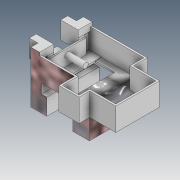
# Autodesk Inventor part: Peça1,61
Saved by Autodesk Inventor 2021 (Build 250183000, 183)
## iProperties
Created: 2020-10-08
Part Number: Peça1,61
Material: Genérico
Document SubType Name: Modeling
Designer: evert
Density: 1 g/cm^3
Appearance: Padrão
Author: evert
Autodesk Inventor part; units mm, degrees
ref_plane "YZ Plane" through (0, 0, 0) normal (1, 0, 0) x (0, 1, 0)
ref_plane "XZ Plane" through (0, 0, 0) normal (0, 1, 0) x (-1, 0, 0)
ref_plane "XY Plane" through (0, 0, 0) normal (0, 0, 1) x (1, 0, 0)
sketch "Esboço2" plane through (0, 0, 0) normal (0, 0, 1) x (1, 0, 0)
  line L0 (0, 0) -> (-5, 0)
  line L1 (-5, 0) -> (-5, -5)
  line L2 (-5, -5) -> (-2, -5)
  line L3 (-2, -5) -> (-2, -15)
  line L4 (-2, -15) -> (-5.6275, -15)
  line L5 (-5.6275, -15) -> (-5.6275, -20)
  line L6 (-5.6275, -20) -> (0, -20)
  line L7 (0, -20) -> (0, -17.5)
  line L8 (0, -17.5) -> (10, -17.5)
  line L9 (10, -17.5) -> (10, -20)
  line L10 (10, -20) -> (15, -20)
  line L11 (15, -20) -> (15, -15)
  line L12 (15, -15) -> (12.5, -15)
  line L13 (12.5, -15) -> (12.5, -5)
  line L14 (12.5, -5) -> (15, -5)
  line L15 (15, 0) -> (15, -5)
  line L16 (15, 0) -> (10, 0)
  line L17 (10, 0) -> (10, -2.5)
  line L18 (10, -2.5) -> (0, -2.5)
  line L19 (0, -2.5) -> (0, 0)
  line L20 (-2.2, -14.8) -> (-2.2, -5.2)
  line L21 (-2.2, -5.2) -> (-4.7, -5.2)
  line L22 (-2.2, -14.8) -> (-4.7, -14.8)
  line L23 (-2.2, -14.8) -> (-5.8275, -14.8)
  line L24 (-5.8275, -14.8) -> (-5.8275, -20)
  line L25 (-5.8275, -20) -> (-5.8275, -20.2)
  line L26 (-5.8275, -20.2) -> (0.2, -20.2)
  line L27 (0.2, -20.2) -> (0.2, -17.7)
  line L28 (0.2, -17.7) -> (9.8, -17.7)
  line L29 (9.8, -17.7) -> (9.8, -18.4636)
  line L30 (9.8, -18.4636) -> (9.8, -20.2)
  line L31 (9.8, -20.2) -> (15.2, -20.2)
  line L32 (15.2, -20.2) -> (15.2, -14.8)
  line L33 (15.2, -14.8) -> (12.7, -14.8)
  line L34 (12.7, -14.8) -> (12.7, -5.2)
  line L35 (12.7, -5.2) -> (15.1265, -5.2)
  line L36 (15.1265, -5.2) -> (15.2, -5.2)
  line L37 (15.2, -5.2) -> (15.2, 0)
  line L38 (-4.7, -5.2) -> (-5.2, -5.2)
  line L39 (-5.2, -5.2) -> (-5.2, 0)
  line L40 (-12.2, 0) -> (-12.2, -24.2)
  line L41 (-12.2, -24.2) -> (22.2, -24.2)
  line L42 (22.2, -24.2) -> (22.2, 0)
  line L43 (15.2, 0) -> (15.2, 0.2)
  line L44 (15.2, 0.2) -> (13.2, 0.2)
  line L45 (22.2, 0) -> (22.2, 1)
  line L46 (22.2, 1) -> (13.2, 1)
  line L47 (13.2, 1) -> (13.2, 0.2)
  line L48 (-12.2, 0) -> (-12.2, 1.2)
  line L49 (-5.2, 0) -> (-5.2, 0.2)
  line L50 (-5.2, 0.2) -> (-3.2, 0.2)
  line L51 (-3.2, 1.2) -> (-12.2, 1.2)
  line L52 (-3.2, 1.2) -> (0, 1.2)
  line L53 (0, 1.2) -> (0, 0.2)
  line L54 (0, 0.2) -> (-3.2, 0.2)
  line L55 (0.5946, -2.5) -> (0.5946, 9.5)
  line L56 (0.5946, 9.5) -> (9.5946, 9.5)
  line L57 (9.5946, 9.5) -> (9.5946, -2.5)
  line L58 (0.5946, -2.5) -> (9.5946, -2.5)
  dimension "d0" = 5
  dimension "d1" = 5
  dimension "d2" = 3
  dimension "d3" = 10
  dimension "d4" = 5
  dimension "d5" = 2.5
  dimension "d6" = 10
  dimension "d7" = 5
  dimension "d8" = 5
  dimension "d9" = 10
  dimension "d11" = 5
  dimension "d12" = 0.2
  dimension "d13" = 0.2
  dimension "d14" = 0.2
  dimension "d15" = 0.2
  dimension "d16" = 0.2
  dimension "d17" = 0.2
  dimension "d19" = 0.2
  dimension "d20" = 0.2
  dimension "d21" = 0.2
  dimension "d22" = 0.2
  dimension "d23" = 0.2
  dimension "d24" = 0.2
  dimension "d25" = 0.2
  dimension "d26" = 0.2
  dimension "d27" = 0.2
  dimension "d28" = 7
  dimension "d29" = 4
  dimension "d30" = 7
  dimension "d31" = 0.2
  dimension "d32" = 2
  dimension "d33" = 1
  dimension "d34" = 0.2
  dimension "d35" = 2
  dimension "d36" = 1
  dimension "d39" = 12
  dimension "d40" = 9
  constraints: 118 end point, 27 perpendicular, 16 point on line, 9 horizontal, 8 vertical, 3 parallel, 1 collinear
  measures "d0" distance of L0.start L0.end
  measures "d1" distance of L0.end L1.end
  measures "d2" distance of L1.end L2.end
  measures "d3" distance of L2.end L3.end
  measures "d4" distance of L4.end L5.end
  measures "d5" distance of L6.end L7.end
  measures "d6" distance of L7.end L8.end
  measures "d7" distance of L9.end L10.end
  measures "d8" distance of L10.end L11.end
  measures "d9" distance of L12.end L13.end
  measures "d11" distance of L15.start L16.end
  measures "d12" distance between parallel lines of L3 L20
  measures "d13" distance between parallel lines of L21 L2
  measures "d14" distance between parallel lines of L4 L22
  measures "d15" distance between parallel lines of L5 L24
  measures "d16" distance between parallel lines of L6 L26
  measures "d17" distance between parallel lines of L7 L27
  measures "d19" distance between parallel lines of L8 L28
  measures "d20" distance between parallel lines of L9 L29
  measures "d21" distance between parallel lines of L31 L10
  measures "d22" distance between parallel lines of L11 L32
  measures "d23" distance between parallel lines of L12 L33
  measures "d24" distance between parallel lines of L34 L13
  measures "d25" distance between parallel lines of L35 L14
  measures "d26" distance between parallel lines of L37 L15
  measures "d27" distance between parallel lines of L1 L39
  measures "d28" distance of L39.end L40.start
  measures "d29" distance from line of L41 L25.end
  measures "d30" distance from line of L42 L31.end
  measures "d31" distance of L37.end L43.end
  measures "d32" distance of L43.end L44.end
  measures "d33" distance of L42.end L45.end
  measures "d34" distance of L39.end L49.end
  measures "d35" distance of L49.end L50.end
  measures "d36" distance between parallel lines of L50 L51
  measures "d39" distance of L55.start L55.end
  measures "d40" distance of L55.end L56.end
extrude "Extrusão1" add sketch "Esboço2" along normal blind 30 contours L22 L23 L24 L25 L26 L27 L28 L29 L30 L31 L32 L33 L34 L35 L36 L37 L43 L44 L47 L46 L45 L42 L41 L40 L48 L51 L52 L53 L54 L50 L49 L39 L38 L21 L20
sketch "Esboço4" plane through (-12.2, -24.2, 0) normal (-1, 0, 0) x (0, 0, 1)
  circle A0 centre (30, 27.7) radius 6 projected
  line L0 (30, 27.7) -> (0, 27.7)
  line L1 (15, 27.7) -> (15, 25.4)
  line L2 (0, 25.4) -> (30, 25.4) projected
  line L3 (0, 27.7) -> (30, 27.7)
  line L4 (30, 27.7) -> (30, 25.4)
  line L5 (30, 25.4) -> (0, 25.4)
  line L6 (0, 25.4) -> (0, 27.7)
  point P0 (0, 24.2)
  constraints: 12 end point, 2 horizontal, 2 midpoint, 2 parallel, 1 perpendicular
extrude "Extrusão2" add sketch "Esboço4" against normal blind 5 contours L0 L4 L2 A0 | A0 L2 L1 L0 | L1 L2 L6 L0 picked at (28.1528, 26.1667)
sketch "Esboço5" plane through (-7.2, -24.2, 0) normal (1, 0, 0) x (0, 0, -1)
  line L0 (-30, 27.7) -> (0, 27.7) projected
  line L1 (0, 27.7) -> (-15, 27.7)
  circle A0 centre (-15, 27.7) radius 1.5
  point P0 (0, 24.2)
  dimension "d48" = 3
  constraints: 2 end point, 1 centre point, 1 coincident, 1 midpoint
  measures "d48" diameter of A0
extrude "Extrusão3" add sketch "Esboço5" along normal blind 13.7
sketch "Esboço6" plane through (-7.2, -24.2, 0) normal (-1, 0, 0) x (0, 0, 1)
  line L0 (13.5, 27.7) -> (16.5, 27.7) projected
  circle A0 centre (15, 27.7) radius 1.5
  point P0 (0, 24.2)
  constraints: 1 centre point, 1 midpoint
extrude "Extrusão4" add sketch "Esboço6" along normal blind 5 contours A0 L0 picked at (15.4855, 27.8197)
sketch "Esboço7" plane through (-12.2, -24.2, 0) normal (-1, 0, 0) x (0, 0, 1)
  circle A0 centre (30, 27.7) radius 6 projected
  line L0 (13.5, 27.7) -> (0, 27.7) projected
  line L1 (30, 33.7) -> (0, 33.7)
  line L2 (0, 33.7) -> (0, 27.7)
  line L3 (0, 27.7) -> (30, 27.7)
  line L4 (30, 27.7) -> (30, 33.7)
  point P0 (0, 24.2)
  constraints: 8 end point, 2 parallel, 1 horizontal, 1 perpendicular, 1 vertical alignment, 1 other
extrude "Extrusão5" add sketch "Esboço7" against normal blind 5 contours L4 L3 A0 | A0 L3 L0 L2 L1 picked at (26.0501, 28.145)
sketch "Esboço8" plane through (-12.2, -24.2, 0) normal (-1, 0, 0) x (0, 0, 1)
  line L0 (30, 33.7) -> (0, 33.7) projected
  line L1 (0, 33.7) -> (0, 35.2)
  line L2 (0, 35.2) -> (30, 35.2)
  line L3 (30, 35.2) -> (30, 33.7)
  line L4 (30, 33.7) -> (0, 33.7)
  line L5 (30, 33.7) -> (30, 25.4) projected
  point P0 (0, 24.2)
  dimension "d55" = 1.5
  constraints: 8 end point, 3 perpendicular, 1 vertical
  measures "d55" distance of L0.end L1.end
extrude "Extrusão6" add sketch "Esboço8" against normal blind 5
sketch "Esboço10" plane through (13.2, 1, 0) normal (0, 1, 0) x (1, 0, 0)
  line L0 (-6.7, -16.5) -> (-6.7, -13.5) projected
  line L1 (-6.7, -15) -> (-6.7, -21.5)
  line L2 (-6.7, -15) -> (-6.7, -8.5)
  line L3 (0, 0) -> (0, -30) projected
  line L4 (0, 0) -> (-13.2, 0)
  line L5 (-3.4, 0) -> (-13, 0) projected
  line L6 (-13.2, 0) -> (-13.2, -8.5)
  line L7 (-13, 0) -> (-13, -30) projected
  line L8 (-13.2, -8.5) -> (0, -8.5)
  line L9 (0, -8.5) -> (0, 0)
  line L10 (2, -30) -> (-3.4, -30) projected
  line L11 (0, -30) -> (0, -21.5)
  line L12 (0, -21.5) -> (-13.2, -21.5)
  line L13 (-13.2, 0) -> (-13.2, -30) projected
  line L14 (-13.2, -21.5) -> (-13.2, -30)
  line L15 (-13.2, -30) -> (0, -30)
  dimension "d58" = 6.5
  dimension "d59" = 6.5
  constraints: 20 end point, 5 perpendicular, 5 point on line, 2 collinear, 1 midpoint, 1 parallel
  measures "d58" distance of L1.start L1.end
  measures "d59" distance of L1.start L2.end
extrude "Extrusão7" add sketch "Esboço10" against normal blind 0.8 contours L12 L3 L10 L15 L7 | L7 L15 L13 L12 | L8 L7 L4 L3 | L8 L6 L4 L7
sketch "Esboço15" plane through (22.2, -24.2, 0) normal (1, 0, 0) x (0, 0, -1)
  line L0 (-30, 25.2) -> (-21.5, 25.2) projected
  line L1 (-30, 25.2) -> (0, 25.2)
  line L2 (0, 25.2) -> (0, 24.2)
  line L3 (0, 24.2) -> (-30, 24.2)
  line L4 (-30, 24.2) -> (-30, 25.2)
  constraints: 8 end point, 2 parallel, 1 horizontal, 1 perpendicular
extrude "Extrusão10" add sketch "Esboço15" along normal blind 3
sketch "Esboço16" plane through (0, 1, 8.5) normal (0, 1, 0) x (1, 0, 0)
  line L0 (22.2, -21.5) -> (25.2, -21.5) projected
  line L1 (25.2, 8.5) -> (23.7, 8.5)
  line L2 (23.7, -21.5) -> (25.2, -21.5)
  line L3 (0, -21.5) -> (25.2, -21.5) projected
  line L4 (-12.2, -21.5) -> (-12.2, 8.5) projected
  line L5 (25.2, -21.5) -> (-12.2, -21.5)
  line L6 (-12.2, -21.5) -> (-12.2, -20.5)
  line L7 (-12.2, -20.5) -> (25.2, -20.5)
  line L8 (25.2, -20.5) -> (25.2, -21.5)
  line L9 (0, 8.5) -> (25.2, 8.5) projected
  line L10 (25.2, 8.5) -> (-12.2, 8.5)
  line L11 (-12.2, 8.5) -> (-12.2, 7.5)
  line L12 (-12.2, 7.5) -> (25.2, 7.5)
  line L13 (25.2, 7.5) -> (25.2, 8.5)
  line L14 (25.2, 8.5) -> (24.2, 8.5)
  line L15 (24.2, 8.5) -> (24.2, -21.5)
  line L16 (24.2, -21.5) -> (25.2, -21.5)
  line L17 (25.2, -21.5) -> (25.2, 8.5)
  point P0 (24.2, 7.5)
  point P1 (24.2, -20.5)
  dimension "d70" = 1
  dimension "d71" = 1
  dimension "d73" = 1
  constraints: 28 end point, 7 parallel, 4 horizontal, 3 perpendicular, 3 point on line, 1 midpoint
  measures "d70" distance between parallel lines of L9 L12
  measures "d71" distance between parallel lines of L7 L3
  measures "d73" distance of L16.end L15.end
extrude "Extrusão11" add sketch "Esboço16" along normal blind 10 contours L3 L5 L4 L7 L15 L0 | L15 L7 L8 L0 | L15 L12 L17 L7 | L15 L1 L13 L12 | L12 L4 L10 L9 L1 L15
sketch "Esboço18" plane through (0, 0, 30) normal (0, 0, 1) x (1, 0, 0)
  line L0 (-12.2, 11) -> (-12.2, -24.2) projected
  line L1 (-12.2, -24.2) -> (22.2, -24.2) projected
  line L2 (-12.2, 11) -> (-11.2, 11)
  line L3 (-11.2, 11) -> (-11.2, -24.2)
  line L4 (-11.2, -24.2) -> (-12.2, -24.2)
  line L5 (-12.2, -24.2) -> (-12.2, 11)
  point P0 (0, 0)
  dimension "d76" = 1
  constraints: 8 end point, 2 parallel, 1 horizontal, 1 perpendicular, 1 point on line
  measures "d76" distance of L3.end L4.end
extrude "Extrusão12" cut sketch "Esboço18" against normal through all
sketch "Esboço20" plane through (0, 1, 8.5) normal (0, 1, 0) x (1, 0, 0)
  line L0 (0, 7.5) -> (0, -20.5) projected
  line L1 (12.7, 8.5) -> (12.7, -21.5) projected
  line L2 (0, 0) -> (12.7, 0)
  line L3 (12.7, 0) -> (12.7, 1)
  line L4 (12.7, 1) -> (0, 1)
  line L5 (0, 1) -> (0, 0)
  line L6 (0, 0) -> (13.2, 0) projected
  line L7 (12.7, 1) -> (13.2, 1)
  line L8 (13.2, 1) -> (13.2, 0)
  line L9 (13.2, 0) -> (12.7, 0)
  line L10 (12.7, 0) -> (12.7, 1)
  line L11 (13.2, 0) -> (13.2, -13) projected
  line L12 (0, -20.5) -> (0, -13) projected
  line L13 (13.2, -13) -> (0, -13)
  line L14 (0, -13) -> (0, -14)
  line L15 (0, -14) -> (13.2, -14)
  line L16 (13.2, -14) -> (13.2, -13)
  point P0 (0, 8.5)
  point P1 (0, -14)
  point P2 (0, -13)
  point P3 (0, 1)
  dimension "d79" = 1
  dimension "d80" = 1
  constraints: 24 end point, 6 parallel, 3 horizontal, 3 perpendicular, 3 point on line
  measures "d79" distance between parallel lines of L4 L2
  measures "d80" distance between parallel lines of L15 L13
extrude "Extrusão13" cut sketch "Esboço20" against normal blind 1 contours L4 L1 L2 L0 | L7 L8 L6 L1 | L13 L1 L15 L0 | L13 L16 L15 L1
sketch "Esboço23" plane through (0, 1, 29) normal (0, 1, 0) x (1, 0, 0)
  line L0 (13.2, 21.5) -> (13.2, 6.5) projected
  line L1 (13.2, 6.5) -> (17.9377, 6.5)
  line L2 (17.9377, 6.5) -> (22.2, 6.5)
  line L3 (22.2, 29) -> (22.2, -1) projected
  line L4 (13.2, 6.5) -> (23.7, 6.5)
  line L5 (13.2, 21.5) -> (0, 21.5) projected
  line L6 (13.2, 21.5) -> (23.7, 21.5)
  line L7 (13.2, 21.5) -> (13.2, 6.5)
  line L8 (23.7, 6.5) -> (23.7, 21.5)
  point P0 (0, 29)
  point P1 (22.2, 21.5)
  point P2 (22.2, 6.5)
  dimension "d91" = 10.5
  constraints: 12 end point, 3 point on line, 2 equal length, 1 horizontal, 1 perpendicular
  measures "d91" distance of L0.end L4.end
extrude "Extrusão16" cut sketch "Esboço23" against normal blind 0.5
sketch "Esboço29" plane through (0, 0.5, 29) normal (0, 1, 0) x (1, 0, 0)
  line L0 (13.2, 6.5) -> (13.2, 21.5) projected
  line L1 (13.2, 21.5) -> (10.2, 21.5)
  line L2 (0, 21.5) -> (23.7, 21.5) projected
  line L3 (10.2, 21.5) -> (10.2, 6.5)
  line L4 (23.7, 6.5) -> (0, 6.5) projected
  line L5 (13.2, 6.5) -> (10.2, 6.5)
  line L6 (10.2, 21.5) -> (13.2, 21.5)
  point P0 (0, 29)
  dimension "d102" = 3
  constraints: 8 end point, 2 perpendicular, 2 point on line, 1 collinear
  measures "d102" distance of L0.end L1.end
extrude "Extrusão20" add sketch "Esboço29" against normal blind 0.5
sketch "Esboço38" plane through (-11.2, -24.2, 30) normal (-1, 0, 0) x (0, 0, 1)
  line L0 (0, 35.2) -> (0, 0) projected
  line L1 (-30, 24.2) -> (0, 24.2) projected
  line L2 (0, 24.2) -> (-30, 24.2)
  line L3 (-30, 35.2) -> (0, 35.2) projected
  line L4 (-25, 35.2) -> (-25, 24.2)
  line L5 (-5, 35.2) -> (-5, 24.2)
  line L6 (-5, 24.2) -> (-10, 24.2)
  line L7 (-7.5, 24.2) -> (-22.5, 24.2) projected
  line L8 (-10, 24.2) -> (-10, 27.2)
  line L9 (-10, 27.2) -> (-20, 27.2)
  line L10 (-20, 27.2) -> (-20, 24.2)
  line L11 (-5, 24.2) -> (-5, 29.2)
  line L12 (-5, 29.2) -> (-8, 29.2)
  line L13 (-8, 29.2) -> (-8, 35.2)
  line L14 (-25, 24.2) -> (-25, 29.2)
  line L15 (-25, 29.2) -> (-22, 29.2)
  line L16 (-22, 29.2) -> (-22, 35.2)
  line L17 (-22, 35.2) -> (-8, 35.2)
  point P0 (-5, 24.2)
  dimension "d128" = 20
  dimension "d129" = 5
  dimension "d130" = 5
  dimension "d131" = 3
  dimension "d132" = 10
  dimension "d133" = 5
  dimension "d134" = 3
  dimension "d135" = 3
  constraints: 28 end point, 12 point on line, 7 perpendicular, 2 collinear, 1 vertical
  measures "d128" distance between parallel lines of L5 L4
  measures "d129" distance between parallel lines of L0 L5
  measures "d130" distance of L5.end L6.end
  measures "d131" distance of L6.end L8.end
  measures "d132" distance of L8.end L9.end
  measures "d133" distance of L5.end L11.end
  measures "d134" distance of L11.end L12.end
  measures "d135" distance of L14.end L15.end
extrude "Extrusão25" cut sketch "Esboço38" against normal blind 5 contours L1 L8 L9 L10 L4 L15 L16 L3 L13 L12 L5
sketch "Esboço39" plane through (-7.2, 1.2, 29) normal (0, 1, 0) x (1, 0, 0)
  line L0 (1, 12.5) -> (13.7, 12.5) projected
  line L1 (1, 12.5) -> (1, 4)
  line L2 (1, 4) -> (0, 4) projected
  line L3 (1, 4) -> (0, 4)
  line L4 (1, 24) -> (1, 19) projected
  line L5 (1, 12.5) -> (1, 24)
  line L6 (1, 24) -> (0, 24)
  line L7 (0, 24) -> (0, 24.1)
  line L8 (0, 28) -> (0, 21) projected
  line L9 (0, 24.1) -> (1.1, 24.1)
  line L10 (0, 4) -> (0, 0) projected
  line L11 (0, 4) -> (0, 3.9)
  line L12 (0, 3.9) -> (1.1, 3.9)
  line L13 (1.1, 3.9) -> (1.1, 24.1)
  point P0 (7.2, 29)
  dimension "d138" = 0.1
  dimension "d139" = 1.1
  dimension "d140" = 0.1
  constraints: 18 end point, 3 point on line, 2 collinear, 2 parallel, 2 perpendicular, 1 vertical
  measures "d138" distance of L6.end L7.end
  measures "d139" distance of L7.end L9.end
  measures "d140" distance of L2.end L11.end
extrude "Extrusão26" add sketch "Esboço39" along normal blind 9.8
sketch "Esboço40" plane through (-11.2, 3, 20) normal (0, 1, 0) x (1, 0, 0)
  line L0 (4, 3.5858) -> (4, 0) projected
  line L1 (5, 3.5858) -> (4, 3.5858) projected
  line L2 (4, 0) -> (5, 0)
  line L3 (5, 0) -> (5, 3.5858)
  line L4 (5, 3.5858) -> (4, 3.5858)
  line L5 (4, 3.5858) -> (4, 0)
  line L6 (4, 6.4142) -> (5, 6.4142) projected
  line L7 (4, 6.4142) -> (5, 6.4142)
  line L8 (5, 6.4142) -> (5, 10)
  line L9 (5, 10) -> (4, 10)
  line L10 (4, 10) -> (4, 6.4142)
  point P0 (11.2, 20)
  constraints: 16 end point, 4 parallel, 2 horizontal, 2 perpendicular
extrude "Extrusão27" add sketch "Esboço40" against normal blind 10
sketch "Esboço41" plane through (-7.2, 1.2, 29) normal (0, 1, 0) x (1, 0, 0)
  line L0 (1, 19) -> (1, 15.4142) projected
  line L1 (1, 19) -> (1.8, 19)
  line L2 (1.3725, 29) -> (1.3725, -1) projected
  line L3 (1, 24) -> (1, 4) projected
  line L4 (1, 9.0006) -> (1.8, 9.0006)
  line L5 (1.8, 19) -> (1.8, 9.0006)
  line L6 (1.8, 9.0006) -> (1.8, 3.2006)
  line L7 (1.8, 3.2006) -> (0, 3.2006)
  line L8 (1.8, 19) -> (1.8, 24.8)
  line L9 (1.8, 24.8) -> (0, 24.8)
  line L10 (0, 28) -> (0, 24.1) projected
  line L11 (0, 24.8) -> (0, 24.1)
  line L12 (1.1, 24.1) -> (0, 24.1) projected
  line L13 (0, 24.1) -> (1.1, 24.1)
  line L14 (0, 3.9) -> (0, 0) projected
  line L15 (0, 3.2006) -> (0, 3.9)
  line L16 (0, 3.9) -> (1.1, 3.9) projected
  line L17 (0, 3.9) -> (1.1, 3.9)
  line L18 (1.1, 3.9) -> (1.1, 9.0006)
  line L19 (1.1, 3.9) -> (1.1, 24.1) projected
  line L20 (1.1, 3.9) -> (1.1, 24.1)
  line L21 (0, 28) -> (0, 24.1) projected
  line L22 (0, 24.1) -> (1.1, 24.1)
  line L23 (0, 24.1) -> (0, 24.8)
  point P0 (7.2, 29)
  point P1 (1.1, 19)
  dimension "d149" = 5.8
  dimension "d150" = 5.8
  constraints: 30 end point, 6 perpendicular, 4 collinear, 3 point on line, 3 vertical, 1 horizontal
  measures "d149" distance of L4.end L6.end
  measures "d150" distance of L1.end L8.end
extrude "Extrusão28" add sketch "Esboço41" along normal blind 9.8
sketch "Esboço42" plane through (-7.2, -24.2, 0) normal (1, 0, 0) x (0, 0, -1)
  line L0 (-22, 35.2) -> (-25, 35.2) projected
  line L1 (-22, 35.2) -> (-22, 29.2)
  line L2 (-22, 29.2) -> (-25, 29.1118)
  line L3 (-25, 25.4) -> (-25, 35.2) projected
  line L4 (-25, 35.2) -> (-25, 35.2) projected
  line L5 (-25, 29.2) -> (-22, 29.2) projected
  line L6 (-25, 35.2) -> (-25, 29.2)
  line L7 (-22, 29.2) -> (-22, 35.2) projected
  line L8 (-25, 35.2) -> (-22, 35.2)
  point P0 (0, 24.2)
  constraints: 8 end point, 1 horizontal, 1 perpendicular, 1 point on line
extrude "Extrusão29" add sketch "Esboço42" along normal blind 1.5 contours L1 L5 L3 L0
sketch "Esboço43" plane through (-7.2, -24.2, 0) normal (1, 0, 0) x (0, 0, -1)
  line L0 (-5, 35.2) -> (-5, 35.4) projected
  line L1 (-8, 35.2) -> (-5, 35.2)
  line L2 (-5, 35.2) -> (-8, 35.2) projected
  line L3 (-8, 35.2) -> (-7.9375, 31.75)
  line L4 (-8, 35.2) -> (-8, 29.2086)
  line L5 (-8, 29.2086) -> (-5, 29.2)
  line L6 (-5, 29.2) -> (-5, 35.2)
  point P0 (0, 24.2)
  constraints: 10 end point, 1 collinear, 1 horizontal, 1 vertical
extrude "Extrusão30" add sketch "Esboço43" along normal blind 1.5
sketch "Esboço44" plane through (-11.2, -24.2, 30) normal (-1, 0, 0) x (0, 0, 1)
  line L0 (-7.5, 24.2) -> (-22.5, 24.2) projected
  line L1 (-20, 27.2) -> (-9.9695, 27.2)
  line L2 (-9.9695, 27.2) -> (-9.9695, 24.2)
  line L3 (-9.9695, 24.2) -> (-20, 24.2)
  line L4 (-20, 24.2) -> (-20, 27.2)
  point P0 (-30, 24.2)
  constraints: 8 end point, 2 parallel, 1 horizontal, 1 perpendicular, 1 point on line
extrude "Extrusão31" add sketch "Esboço44" along normal blind 5
sketch "Esboço45" plane through (-11.2, -24.2, 30) normal (-1, 0, 0) x (0, 0, 1)
  line L0 (-8, 35.2) -> (-8, 29.2) projected
  line L1 (-8, 29.2) -> (-8, 39.2)
  line L2 (-8, 39.2) -> (0, 39.2)
  line L3 (-8, 35.2) -> (0, 35.2) projected
  line L4 (0, 39.2) -> (0, 35.2)
  line L5 (0, 35.2) -> (-8, 35.2)
  line L6 (-30, 35.2) -> (-22, 35.2) projected
  line L7 (-22, 35.2) -> (-22, 39.2)
  line L8 (-22, 39.2) -> (-30, 39.2)
  line L9 (-30, 39.2) -> (-30, 35.2)
  line L10 (-8, 29.2) -> (-5, 29.2) projected
  line L11 (-8, 29.2) -> (0, 29.2)
  line L12 (0, 29.2) -> (0, 39.2)
  line L13 (-22, 35.2) -> (-22, 29.2086) projected
  line L14 (-22, 35.2) -> (-22, 29.2086)
  line L15 (-22, 29.2086) -> (-30, 29.2)
  line L16 (-30, 0) -> (-30, 35.2) projected
  line L17 (-30, 39.2) -> (-30, 29.2)
  point P0 (-30, 24.2)
  dimension "d157" = 10
  constraints: 24 end point, 4 collinear, 3 perpendicular, 2 horizontal, 2 point on line, 1 vertical
  measures "d157" distance of L0.end L1.end
extrude "Extrusão32" add sketch "Esboço45" along normal blind 5
sketch "Esboço46" plane through (-11.2, -24.2, 30) normal (1, 0, 0) x (0, 0, -1)
  line L0 (0, 39.2) -> (8, 39.2) projected
  line L1 (8, 39.2) -> (8, 35.2) projected
  line L2 (0, 39.2) -> (8, 39.2)
  line L3 (8, 39.2) -> (8, 35.2)
  line L4 (0, 35.2) -> (0, 39.2) projected
  line L5 (8, 35.2) -> (0, 35.2)
  line L6 (0, 35.2) -> (0, 39.2)
  line L7 (22, 29.2086) -> (22, 39.2) projected
  line L8 (22, 39.2) -> (30, 39.2)
  line L9 (30, 35.2) -> (22, 35.2) projected
  line L10 (30, 39.2) -> (30, 35.2)
  line L11 (30, 35.2) -> (22, 35.2)
  line L12 (22, 35.2) -> (22, 39.2)
  point P0 (30, 24.2)
  constraints: 16 end point, 3 collinear, 3 perpendicular, 2 horizontal
extrude "Extrusão33" add sketch "Esboço46" along normal blind 5
sketch "Esboço47" plane through (-16.2, -24.2, 30) normal (-1, 0, 0) x (0, 0, 1)
  line L0 (0, 29.2) -> (-5, 29.2) projected
  line L1 (-8, 29.2) -> (-5, 29.2)
  line L2 (-8, 29.2) -> (-4, 29.2)
  line L3 (-4, 29.2) -> (-4, 39.2)
  line L4 (0, 39.2) -> (-8, 39.2) projected
  line L5 (0, 39.2) -> (-4, 39.2)
  line L6 (0, 29.2) -> (0, 39.2) projected
  line L7 (0, 39.2) -> (0, 29.2)
  line L8 (0, 29.2) -> (-4, 29.2)
  line L9 (-25, 29.2) -> (-22, 29.2) projected
  line L10 (-22, 29.2) -> (-26, 29.2043)
  line L11 (-22, 29.2086) -> (-30, 29.2) projected
  line L12 (-26, 29.2043) -> (-26, 39.2)
  line L13 (-30, 39.2) -> (-22, 39.2) projected
  line L14 (-30, 39.2) -> (-26, 39.2)
  line L15 (-30, 35.2) -> (-30, 39.2) projected
  line L16 (-30, 39.2) -> (-30, 29.2086)
  line L17 (-30, 29.2086) -> (-26, 29.2043)
  point P0 (-30, 24.2)
  dimension "d163" = 4
  constraints: 22 end point, 5 collinear, 3 midpoint, 3 point on line, 1 perpendicular
  measures "d163" distance of L1.start L2.end
extrude "Extrusão34" cut sketch "Esboço47" against normal blind 5
sketch "Esboço48" plane through (-16.2, 5.0043, 4) normal (0, 1, 0.0011) x (1, 0, 0)
  line L0 (5, 4) -> (5, 4.0107) projected
  line L1 (5, 0) -> (5, 4) projected
  line L2 (5, 4.0107) -> (5, 0)
  line L3 (5, 0.0107) -> (0, 0.0107) projected
  line L4 (5, 0) -> (0, 0.0107)
  line L5 (0, 4) -> (5, 4) projected
  line L6 (0.0086, 4.0107) -> (5, 4.0107)
  line L7 (0, 0.0107) -> (0, 0) projected
  line L8 (0, 0) -> (-1.8529, 0)
  line L9 (-1.8529, 0) -> (-1.8529, 4)
  line L10 (-1.8529, 4) -> (0, 4)
  point P0 (16.2, 3.9946)
  constraints: 12 end point, 2 perpendicular, 1 horizontal, 1 vertical, 1 vertical alignment, 2 other
extrude "Extrusão35" cut sketch "Esboço48" against normal blind 5 contours L3 L7 L8 L9 L10 L5 L1
sketch "Esboço50" plane through (22.2, -24.2, 0) normal (0, -1, 0) x (1, 0, 0)
  line L0 (-28.4, 0) -> (-38.4, 0) projected
  line L1 (0, 30) -> (-33.4, 30)
  line L2 (-33.4, 30) -> (-33.4, 0)
  line L3 (-33.4, 0) -> (0, 0)
  line L4 (0, 0) -> (0, 30)
  point P0 (-22.2, 0)
  constraints: 8 end point, 2 parallel, 1 horizontal, 1 perpendicular
extrude "Extrusão36" cut sketch "Esboço50" against normal blind 9.5
sketch "Esboço51" plane through (25.2, 11, 30) normal (0, 1, 0) x (1, 0, 0)
  line L0 (-36.4, 0) -> (-27.4, 0) projected
  line L1 (-31.407, 0) -> (0, 0)
  line L2 (0, 0) -> (0, 30)
  line L3 (0, 30) -> (-31.407, 30)
  line L4 (-31.407, 30) -> (-31.407, 0)
  line L5 (0, 30) -> (-31.407, 30)
  line L6 (-31.407, 30) -> (-31.407, 50)
  line L7 (-31.407, 50) -> (0, 50)
  line L8 (0, 50) -> (0, 30)
  point P0 (-25.2, 30)
  dimension "d172" = 20
  constraints: 16 end point, 4 parallel, 2 horizontal, 2 perpendicular, 2 point on line
  measures "d172" distance of L5.end L6.end
extrude "Extrusão37" cut sketch "Esboço51" against normal blind 1.2 contours L4 L3 L2 L1 L0
sketch "Esboço52" plane through (0, 1, 29) normal (0, 1, 0) x (1, 0, 0)
  line L0 (10.2, 21.5) -> (13.2, 21.5) projected
  line L1 (10.2, 6.5) -> (10.2, 21.5) projected
  line L2 (10.2, 21.5) -> (10.2, 6.5)
  line L3 (13.2, 6.5) -> (10.2, 6.5) projected
  line L4 (10.2, 6.5) -> (10.2, 14)
  line L5 (10.2, 14) -> (0, 14)
  line L6 (0, 21.5) -> (0, 6.5) projected
  line L7 (10.2, 14) -> (10.2, 21.5)
  line L8 (10.2, 14) -> (10.2, 24.5)
  line L9 (10.2, 14) -> (10.2, 3.5)
  line L10 (10.2, 3.5) -> (0, 3.5)
  line L11 (0, 28) -> (0, 0) projected
  line L12 (0, 3.5) -> (0, 24.5)
  line L13 (0, 21.5) -> (0, 28) projected
  line L14 (0, 24.5) -> (10.2, 24.5)
  point P0 (0, 29)
  point P1 (10.2, 6.5)
  point P2 (10.2, 21.5)
  dimension "d175" = 10.5
  dimension "d176" = 10.5
  dimension "d177" = 21
  constraints: 18 end point, 3 point on line, 2 midpoint, 1 collinear, 1 perpendicular, 1 vertical
  measures "d175" distance of L4.end L8.end
  measures "d176" distance of L4.end L9.end
  measures "d177" distance of L10.end L12.end
extrude "Extrusão38" cut sketch "Esboço52" against normal blind 10
sketch "Esboço53" plane through (0, 0.5, 29) normal (0, 1, 0) x (1, 0, 0)
  line L0 (10.2, 6.5) -> (13.2, 6.5) projected
  line L1 (23.7, 21.5) -> (23.7, 6.5) projected
  line L2 (10.2, 6.5) -> (23.7, 6.5)
  line L3 (23.7, 6.5) -> (23.7, 21.5)
  line L4 (23.7, 21.5) -> (10.2, 21.5)
  line L5 (10.2, 21.5) -> (10.2, 6.5)
  point P0 (0, 29)
  point P1 (13.2, 6.5)
  constraints: 8 end point, 2 parallel, 1 horizontal, 1 perpendicular
extrude "Extrusão39" add sketch "Esboço53" along normal blind 0.5
sketch "Esboço56" plane through (25.2, 9.8, 30) normal (0, 1, 0) x (1, 0, 0)
  line L0 (0, 0) -> (-31.407, 0) projected
  line L1 (-12.5, 30) -> (-12.5, 0) projected
  line L2 (0, 0) -> (-12.5, 0)
  line L3 (-12.5, 0) -> (-12.5, 28.9999)
  line L4 (-12.5, 28.9999) -> (0, 28.9999)
  line L5 (0, 28.9999) -> (0, 0)
  point P0 (-25.2, 30)
  constraints: 8 end point, 2 parallel, 1 horizontal, 1 perpendicular, 1 point on line
extrude "Extrusão40" cut sketch "Esboço56" against normal blind 8.8
sketch "Esboço57" plane through (-5.4, 1.2, 25.7994) normal (1, 0, 0) x (0, 0, -1)
  circle A0 centre (10.7994, 2.3) radius 1.5 projected
  line L0 (10.7994, 0.8) -> (10.7994, 2.3)
  line L1 (10.7994, 2.3) -> (10.7994, 5.3)
  circle A1 centre (10.7994, 5.3) radius 1.5
  line L2 (12.2994, 2.3) -> (12.2994, 5.3)
  line L3 (9.2994, 2.3) -> (9.2994, 5.3)
  point P0 (25.7994, -1.2)
  dimension "d187" = 3
  dimension "d188" = 3
  constraints: 8 end point, 5 point on circle, 2 tangent, 2 vertical, 1 centre point, 1 coincident, 1 parallel, 1 point on line
  measures "d187" distance of L0.end L1.end
  measures "d188" diameter of A1
extrude "Extrusão41" add sketch "Esboço57" along normal blind 12.2 contours A1
sketch "Esboço58" plane through (6.5, 3.5, 15) normal (1, 0, 0) x (0, 0, -1)
  circle A0 centre (0, 0) radius 1.5
  point P0 (15, -3.5)
  constraints: 1 centre point
extrude "Extrusão42" cut sketch "Esboço58" against normal blind 11.9
sketch "Esboço59" plane through (0, 1, 1) normal (0, 1, 0) x (1, 0, 0)
  line L0 (10.2, -3.5) -> (10.2, -24.5) projected
  line L1 (10.2, -24.5) -> (11.2, -24.5)
  line L2 (11.2, -24.5) -> (11.2, -3.5)
  line L3 (11.2, -3.5) -> (10.2, -3.5)
  line L4 (10.2, -3.5) -> (10.2, -24.5)
  point P0 (0, 1)
  dimension "d193" = 1
  constraints: 8 end point, 2 parallel, 1 horizontal, 1 perpendicular
  measures "d193" distance of L2.end L3.end
extrude "Extrusão43" cut sketch "Esboço59" against normal blind 1
sketch "Esboço61" plane through (6.8, 6.5, 15) normal (1, 0, 0) x (0, 0, -1)
  circle A0 centre (0, 0) radius 1.5 projected
  circle A1 centre (0, 0) radius 1.5
  point P0 (15, -6.5)
  constraints: 1 centre point, 1 coincident
extrude "Extrusão44" cut sketch "Esboço61" against normal blind 1.8
sketch "Esboço62" plane through (25.2, 9.8, 30) normal (0, 1, 0) x (1, 0, 0)
  line L0 (-31.4, 30) -> (-31.4, 22) projected
  line L1 (-31.4, 29.0001) -> (-31.4, 30)
  line L2 (-31.4, 30) -> (0.1, 30)
  line L3 (0.1, 30) -> (0.1, 22.04)
  line L4 (0.1, 30) -> (-0.9, 30)
  line L5 (-3, 30) -> (0, 30) projected
  line L6 (-0.9, 30) -> (-0.9, 21.04)
  line L7 (-0.9, 21.04) -> (14, 21.04)
  line L8 (0.1, 22.04) -> (15, 22.04)
  line L9 (15, 22.04) -> (15, -2.96)
  line L10 (14, 21.04) -> (14, -1.96)
  line L11 (15, -2.96) -> (0.1, -2.96)
  line L12 (14, -1.96) -> (-0.9, -1.96)
  line L13 (-0.9, -1.96) -> (-0.9, -7.96)
  line L14 (0.1, -2.96) -> (0.1, -8.96)
  line L15 (0.1, -8.96) -> (-11.5, -8.96)
  line L16 (-0.9, -7.96) -> (-10.5, -7.96)
  line L17 (-11.5, -8.96) -> (-11.5, 1)
  line L18 (-10.5, -7.96) -> (-10.5, 1)
  line L19 (-10, 0) -> (-12.5, 0) projected
  line L20 (-25.2, 1) -> (-12.5, 1) projected
  line L21 (-10.5, 1) -> (-12.5, 1)
  line L22 (-12.5, 30) -> (-12.5, 0) projected
  line L23 (-12.5, 1) -> (-12.5, 0)
  line L24 (-12.5, 0) -> (-10.5, 0)
  point P0 (-25.2, 30)
  point P1 (-11.5, 0)
  point P2 (-0.9, 30)
  dimension "d198" = 31.5
  dimension "d199" = 7.96
  dimension "d200" = 1
  dimension "d201" = 8.96
  dimension "d202" = 14.9
  dimension "d203" = 14.9
  dimension "d204" = 25
  dimension "d205" = 23
  dimension "d206" = 14.9
  dimension "d207" = 14.9
  dimension "d208" = 6
  dimension "d209" = 6
  dimension "d210" = 11.6
  dimension "d211" = 9.6
  dimension "d212" = 9.96
  dimension "d213" = 8.96
  constraints: 40 end point, 7 horizontal, 7 vertical, 4 point on line, 1 collinear, 1 perpendicular
  measures "d198" distance of L0.start L2.end
  measures "d199" distance of L2.end L3.end
  measures "d200" distance of L2.end L4.end
  measures "d201" distance of L4.end L6.end
  measures "d202" distance of L6.end L7.end
  measures "d203" distance of L3.end L8.end
  measures "d204" distance of L8.end L9.end
  measures "d205" distance of L7.end L10.end
  measures "d206" distance of L9.end L11.end
  measures "d207" distance of L10.end L12.end
  measures "d208" distance of L12.end L13.end
  measures "d209" distance of L11.end L14.end
  measures "d210" distance of L14.end L15.end
  measures "d211" distance of L13.end L16.end
  measures "d212" distance of L15.end L17.end
  measures "d213" distance of L16.end L18.end
extrude "Extrusão45" add sketch "Esboço62" against normal blind 8.8 contours L21 L17 L19 L22 | L2 L3 L8 L9 L11 L14 L15 L17 L19 L18 L16 L13 L12 L10 L7 L6 | L21 L18 L19 L17
sketch "Esboço63" plane through (25.2, 9.8, 30) normal (0, 1, 0) x (1, 0, 0)
  line L0 (-31.4, 8) -> (-31.4, 0) projected
  line L1 (-31.407, 1) -> (-10.5, 1) projected
  line L2 (-31.4, 0) -> (-10.5, 0)
  line L3 (-10.5, 0) -> (-10.5, 1)
  line L4 (-10.5, 1) -> (-31.4, 1)
  line L5 (-31.4, 1) -> (-31.4, 0)
  line L6 (-11.5, 0) -> (-11.5, -8.96) projected
  line L7 (-10.5, 1) -> (-11.5, 1)
  line L8 (-11.5, 1) -> (-11.5, -8.96)
  line L9 (-11.5, -8.96) -> (-10.5, -8.96)
  line L10 (-10.5, -8.96) -> (-10.5, 1)
  line L11 (-11.5, -8.96) -> (0.1, -8.96) projected
  line L12 (-10.5, -7.96) -> (-0.9, -7.96) projected
  line L13 (-11.5, -8.96) -> (-0.9, -8.96)
  line L14 (-0.9, -8.96) -> (-0.9, -7.96)
  line L15 (-0.9, -7.96) -> (-11.5, -7.96)
  line L16 (-11.5, -7.96) -> (-11.5, -8.96)
  line L17 (-0.9, -1.96) -> (14, -1.96) projected
  line L18 (-0.9, -8.96) -> (0.1, -8.96)
  line L19 (0.1, -8.96) -> (0.1, -1.96)
  line L20 (0.1, -1.96) -> (-0.9, -1.96)
  line L21 (-0.9, -1.96) -> (-0.9, -8.96)
  line L22 (-0.9, -7.96) -> (-0.9, -1.96) projected
  line L23 (15, 22.04) -> (15, -2.96) projected
  line L24 (-0.9, -1.96) -> (15, -1.96)
  line L25 (15, -1.96) -> (15, -2.96)
  line L26 (15, -2.96) -> (-0.9, -2.96)
  line L27 (-0.9, -2.96) -> (-0.9, -1.96)
  line L28 (15, -2.96) -> (0.1, -2.96) projected
  line L29 (0.1, 22.04) -> (15, 22.04) projected
  line L30 (15, -2.96) -> (14, -2.96)
  line L31 (14, -2.96) -> (14, 22.04)
  line L32 (14, 22.04) -> (15, 22.04)
  line L33 (15, 22.04) -> (15, -2.96)
  line L34 (0, 21.04) -> (-0.9, 21.04) projected
  line L35 (15, 22.04) -> (-0.9, 22.04)
  line L36 (-0.9, 22.04) -> (-0.9, 21.04)
  line L37 (-0.9, 21.04) -> (15, 21.04)
  line L38 (15, 21.04) -> (15, 22.04)
  line L39 (-0.9, 28.9999) -> (-0.9, 21.04) projected
  line L40 (0.1, 30) -> (0.1, 22.04) projected
  line L41 (-0.9, 21.04) -> (0.1, 21.04)
  line L42 (0.1, 21.04) -> (0.1, 30)
  line L43 (0.1, 30) -> (-0.9, 30)
  line L44 (-0.9, 30) -> (-0.9, 21.04)
  line L45 (-31.407, 29) -> (-31.407, 30) projected
  line L46 (0.1, 30) -> (-31.407, 30)
  line L47 (-31.407, 30) -> (-31.407, 29)
  line L48 (-31.407, 29) -> (0.1, 29)
  line L49 (0.1, 29) -> (0.1, 30)
  point P0 (-25.2, 30)
  point P1 (-0.9, 29)
  point P2 (14, 21.04)
  dimension "d216" = 1
  dimension "d217" = 1
  constraints: 72 end point, 18 parallel, 9 horizontal, 9 perpendicular, 2 point on line
  measures "d216" distance of L20.end L19.end
  measures "d217" distance of L31.end L32.end
extrude "Extrusão46" add sketch "Esboço63" along normal blind 3.2
sketch "Esboço64" plane through (25.2, 1, 30) normal (0, -1, 0) x (1, 0, 0)
  line L0 (0.1, -30) -> (-31.4, -30) projected
  line L1 (0, -30) -> (0.1, -30)
  line L2 (0.1, -22.04) -> (15, -22.04) projected
  line L3 (0.1, -30) -> (0.1, -22.04)
  line L4 (15, -22.04) -> (15, 2.96) projected
  line L5 (15, -22.04) -> (15, 2.96)
  line L6 (15, 2.96) -> (0.1, 2.96)
  line L7 (14, 1.96) -> (-0.9, 1.96) projected
  line L8 (0.1, 2.96) -> (0.1, 8.96) projected
  line L9 (0.1, 2.96) -> (0.1, 8.96)
  line L10 (-11.5, 8.96) -> (-11.5, 0) projected
  line L11 (0.1, 8.96) -> (-11.5, 8.96)
  line L12 (-10.5, 0) -> (-11.5, 0) projected
  line L13 (-11.5, 0) -> (-10.5, 0)
  line L14 (-10.5, 0) -> (-11.5, 0)
  line L15 (-10.5, 0) -> (-10.5, 7.96) projected
  line L16 (0, 0) -> (-10.5, 0) projected
  line L17 (-10.5, 0) -> (0, 0)
  line L18 (0, 0) -> (0, -30) projected
  line L19 (0, -30) -> (0, -21.04) projected
  line L20 (0, 0) -> (0, -30)
  point P0 (-25.2, -30)
  constraints: 20 end point, 5 collinear, 3 perpendicular, 1 horizontal, 1 parallel, 1 point on line
extrude "Extrusão47" add sketch "Esboço64" along normal blind 1
